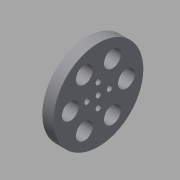
# Autodesk Inventor part: ShoulderGearYZ
Saved by Autodesk Inventor 2017 (Build 210142000, 142)
## iProperties
Created: 2017-05-07
Part Number: ShoulderGearYZ
Material: Generic
Document SubType Name: Modeling
Designer: zallen
Density: 1 g/cm^3
Appearance: Default
Author: zallen
Autodesk Inventor part; units mm, degrees
ref_plane "YZ Plane" through (0, 0, 0) normal (1, 0, 0) x (0, 1, 0)
ref_plane "XZ Plane" through (0, 0, 0) normal (0, 1, 0) x (-1, 0, 0)
ref_plane "XY Plane" through (0, 0, 0) normal (0, 0, 1) x (1, 0, 0)
sketch "Sketch1" plane through (0, 0, 0) normal (1, 0, 0) x (0, 1, 0)
  circle A0 centre (0, 0) radius 50.8
  circle A1 centre (0, 0) radius 3.175
  circle A2 centre (0, -31.75) radius 9.525
  line L0 (0, 0) -> (0, -74.7092) construction
  circle A3 centre (27.4963, -15.875) radius 9.525
  circle A4 centre (27.4963, 15.875) radius 9.525
  circle A5 centre (0, 31.75) radius 9.525
  circle A6 centre (-27.4963, 15.875) radius 9.525
  circle A7 centre (-27.4963, -15.875) radius 9.525
  circle A8 centre (0, -12.7) radius 3.175
  circle A9 centre (12.7, 0) radius 3.175
  circle A10 centre (0, 12.7) radius 3.175
  circle A11 centre (-12.7, 0) radius 3.175
  dimension "d0" = 101.6
  dimension "d1" = 6.35
  dimension "d2" = 19.05
  dimension "d3" = 31.75
  dimension "d6" = 360
  dimension "d16" = 6.35
  dimension "d17" = 12.7
  dimension "d24" = 360
  constraints: 12 centre point, 2 coincident, 2 end point, 2 point on line, 1 vertical, 22 other
  measures "d0" diameter of A0
  measures "d1" diameter of A1
  measures "d2" diameter of A2
  measures "d3" distance of A2.centre point (0, 0)
  measures "d16" diameter of A8
  measures "d17" distance of point (0, 0) A8.centre
extrude "Extrusion3" add sketch "Sketch1" along normal blind 12.7
sketch "Sketch4" plane through (0, 0, 0) normal (-1, 0, 0) x (0, 0, 1)
  circle A0 centre (0, 0) radius 6.35
  circle A1 centre (0, 0) radius 3.175
  dimension "d28" = 12.7
  dimension "d31" = 6.35
  constraints: 2 centre point, 2 coincident
  measures "d28" diameter of A0
  measures "d31" diameter of A1
extrude "Extrusion5" add sketch "Sketch4" along normal blind 6.35
sketch "Sketch5" plane through (0, 0, 0) normal (0, 1, 0) x (-1, 0, 0)
  circle A0 centre (3.175, 0) radius 1.5875
  line L0 (0, 0) -> (21.9133, 0) construction
  line L1 (6.35, -6.35) -> (6.35, 6.35) construction
  dimension "d34" = 3.175
  dimension "d35" = 3.175
  constraints: 2 end point, 1 centre point, 1 horizontal, 1 point on line
  measures "d34" diameter of A0
  measures "d35" distance from line of L1 A0.centre
extrude "Extrusion6" cut sketch "Sketch5" along normal through all
body "Solid3"
